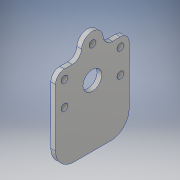
# Autodesk Inventor part: CaseSheet_2019
Saved by Autodesk Inventor 2019.4 (Build 234330000, 330)
## iProperties
Created: 2020-02-07
Part Number: CaseSheet_2019
Material: Aluminum 6061
Document SubType Name: Modeling
Designer: Paul Lefeuvre
Density: 2.7 g/cm^3
Appearance: Aluminum - Flat
Author: Paul Lefeuvre
Autodesk Inventor part; units mm, degrees
ref_plane "YZ Plane" through (0, 0, 0) normal (1, 0, 0) x (0, 1, 0)
ref_plane "XZ Plane" through (0, 0, 0) normal (0, 1, 0) x (-1, 0, 0)
ref_plane "XY Plane" through (0, 0, 0) normal (0, 0, 1) x (1, 0, 0)
sketch "Sketch1" plane through (0, 0, 0) normal (1, 0, 0) x (0, 1, 0)
  circle A0 centre (0, 0) radius 10.1
  circle A1 centre (16, 30) radius 3.6
  circle A2 centre (-10, 30) radius 3.6
  circle A3 centre (16, -30) radius 3.6
  circle A4 centre (-10, -30) radius 3.6
  line L0 (25.5, 30) -> (25.5, -30)
  line L1 (16, -39.5) -> (-46, -39.5)
  line L2 (-66, -19.5) -> (-66, 19.5)
  line L3 (-46, 39.5) -> (16, 39.5)
  arc A5 (-46, 39.5) -> (-66, 19.5) centre (-46, 19.5) ccw
  arc A6 (-66, -19.5) -> (-46, -39.5) centre (-46, -19.5) ccw
  arc A7 (25.5, 30) -> (16, 39.5) centre (16, 30) ccw
  arc A8 (16, -39.5) -> (25.5, -30) centre (16, -30) ccw
  line L4 (0, 0) -> (34, 0) construction
  circle A9 centre (34, 0) radius 3.6
  arc A10 (34.8056, -11.572) -> (34.8056, 11.572) centre (34, 0) ccw
  arc A11 (25.5, 21.5479) -> (34.8056, 11.572) centre (35.5, 21.5479) ccw
  arc A12 (34.8056, -11.572) -> (25.5, -21.5479) centre (35.5, -21.5479) ccw
  dimension "d0" = 20.2
  dimension "d1" = 7.2
  dimension "d2" = 30
  dimension "d3" = 16
  dimension "d4" = 7.2
  dimension "d5" = 10
  dimension "d6" = 30
  dimension "d7" = 7.2
  dimension "d8" = 7.2
  dimension "d9" = 30
  dimension "d10" = 16
  dimension "d11" = 10
  dimension "d12" = 30
  dimension "d13" = 9.5
  dimension "d14" = 9.5
  dimension "d15" = 9.5
  dimension "d16" = 66
  dimension "d17" = 20
  dimension "d18" = 9.5
  dimension "d21" = 7.2
  dimension "d22" = 34
  dimension "d23" = 11.6
  dimension "d24" = 10
  dimension "d25" = 10
  constraints: 14 point on circle, 13 centre point, 12 tangent, 10 end point, 3 coincident, 3 perpendicular, 2 equal radius, 2 point on line, 1 horizontal, 1 vertical
  measures "d0" diameter of A0
  measures "d1" diameter of A1
  measures "d2" vertical distance of A1.centre point (0, 0)
  measures "d3" horizontal distance of A1.centre point (0, 0)
  measures "d4" diameter of A2
  measures "d5" horizontal distance of A2.centre L4.start
  measures "d6" vertical distance of point (0, 0) A2.centre
  measures "d7" diameter of A3
  measures "d8" diameter of A4
  measures "d9" vertical distance of point (0, 0) A3.centre
  measures "d10" horizontal distance of point (0, 0) A3.centre
  measures "d11" horizontal distance of point (0, 0) A4.centre
  measures "d12" vertical distance of point (0, 0) A4.centre
  measures "d13" distance from line of L0 A3.centre
  measures "d14" distance from line of L1 A3.centre
  measures "d15" distance from line of A1.centre L3
  measures "d16" distance from line of L2 L4.start
  measures "d17" radius of A5
  measures "d18" radius of A7
  measures "d21" diameter of A9
  measures "d22" distance of L4.start L4.end
  measures "d23" radius of A10
  measures "d24" radius of A11
  measures "d25" radius of A12
extrude "Extrusion1" add sketch "Sketch1" along normal blind 5
equation "\"d6\" = d2"
equation "\"d9\" = d2"
equation "\"d10\" = d3"
equation "\"d11\" = d5"
equation "\"d12\" = d2"
equation "\"d14\" = d13"
equation "\"d15\" = d13"
equation "\"d18\" = d13"
body "Solid1"
